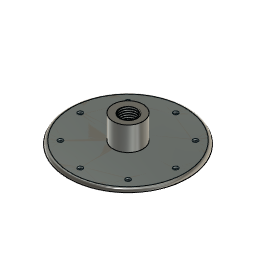
Top Panel Mount v4 (Autodesk Fusion 360 design; units mm, degrees)
Autodesk Fusion 360 part; units mm, degrees
sketch "Sketch1" plane through (0, 0, 0) normal (0, 0, 1) x (1, 0, 0)
  circle A0 centre (0, 0) radius 100
  circle A1 centre (0, 0) radius 80
  circle A2 centre (80, 0) radius 1.5
  circle A3 centre (56.5685, 56.5685) radius 1.5
  circle A4 centre (0, 0) radius 80
  circle A5 centre (0, 80) radius 1.5
  circle A6 centre (0, 0) radius 80
  circle A7 centre (-56.5685, 56.5685) radius 1.5
  circle A8 centre (0, 0) radius 80
  circle A9 centre (-80, 0) radius 1.5
  circle A10 centre (0, 0) radius 80
  circle A11 centre (-56.5685, -56.5685) radius 1.5
  circle A12 centre (0, 0) radius 80
  circle A13 centre (0, -80) radius 1.5
  circle A14 centre (0, 0) radius 80
  circle A15 centre (56.5685, -56.5685) radius 1.5
  circle A16 centre (0, 0) radius 80
  dimension "d1" = 200
  dimension "d4" = 160
  dimension "d5" = 3
  dimension "d7" = 360
  constraint coincident A0.centre A1.centre
  constraint concentric A0 A1
  constraint coincident A1 A2.centre
  measures "d1" diameter of A0
  measures "d4" diameter of A1
  measures "d5" diameter of A2
extrude "Extrude1" add sketch "Sketch1" along normal blind 5 contours A0 | A1 A2 A3 A4 A5 A6 A7 A8 A9 A10 A11 A12 A13 A14 A15 A16
fillet "Fillet1" radius 5 1 edges at (-93.2327, -36.1615, 5)
sketch "Sketch2" plane through (0, 0, 5) normal (0, 0, 1) x (-1, 0, 0)
  circle A0 centre (56.5685, 56.5685) radius 1.5
  circle A1 centre (-56.5685, -56.5685) radius 1.5
  circle A2 centre (0, 80) radius 1.5
  circle A3 centre (-80, 0) radius 1.5
  circle A4 centre (0, -80) radius 1.5
  circle A5 centre (80, 0) radius 1.5
  circle A6 centre (56.5685, -56.5685) radius 1.5
  circle A7 centre (-56.5685, 56.5685) radius 1.5
  circle A8 centre (0, 0) radius 95
  circle A9 centre (-80, 0) radius 4
  circle A10 centre (-56.5685, -56.5685) radius 4
  circle A11 centre (-56.5685, -56.5685) radius 1.5
  circle A12 centre (0, -80) radius 4
  circle A13 centre (0, -80) radius 1.5
  circle A14 centre (56.5685, -56.5685) radius 4
  circle A15 centre (56.5685, -56.5685) radius 1.5
  circle A16 centre (80, 0) radius 4
  circle A17 centre (80, 0) radius 1.5
  circle A18 centre (56.5685, 56.5685) radius 4
  circle A19 centre (56.5685, 56.5685) radius 1.5
  circle A20 centre (0, 80) radius 4
  circle A21 centre (0, 80) radius 1.5
  circle A22 centre (-56.5685, 56.5685) radius 4
  circle A23 centre (-56.5685, 56.5685) radius 1.5
  dimension "d9" = 8
  dimension "d11" = 360
  constraint concentric A3 A9
  measures "d9" diameter of A9
extrude "Extrude2" cut sketch "Sketch2" against normal blind 3 contours A4 A13 | A9 | A10 | A12 | A14 | A16 | A18 | A20 | A22
sketch "Sketch3" plane through (0, 0, 5) normal (0, 0, 1) x (-1, 0, 0)
  circle A0 centre (0, -80) radius 4
  circle A1 centre (0, 80) radius 4
  circle A2 centre (-56.5685, 56.5685) radius 4
  circle A3 centre (56.5685, -56.5685) radius 4
  circle A4 centre (-56.5685, -56.5685) radius 4
  circle A5 centre (56.5685, 56.5685) radius 4
  circle A6 centre (-80, 0) radius 4
  circle A7 centre (80, 0) radius 4
  circle A8 centre (0, 0) radius 95
sketch "Sketch4" plane through (0, 0, 5) normal (0, 0, 1) x (-1, 0, 0)
  circle A0 centre (0, 0) radius 15
  circle A1 centre (0, 0) radius 25
  dimension "d14" = 30
  dimension "d15" = 50
  constraint coincident A0.centre A1.centre
  constraint concentric A0 A1
  measures "d14" diameter of A0
  measures "d15" diameter of A1
extrude "Extrude3" add sketch "Sketch4" along normal blind 40
thread "Thread1" "ISO Metric profile 30.0 M30x3.5 6H" major diameter 30.3925 minor diameter 26.491 pitch 3.5 angle 60 modelled left hand crest width 0.9556 on face at (-14.9814, 0.7477, 31.6667) crest through (-13.2455, 0, 5.875)
